Autodesk Fusion 360 part; units mm, degrees
(part 25 of 25)
sketch "Sketch2 (2)" plane through (0, 0, -3) normal (0, 0, -1) x (1, 0, 0) in component "grub screw"
  circle A0 centre (0, 0) radius 1.3
  line L0 (0.6928, 0.4) -> (0, 0.8)
  line L1 (0, 0.8) -> (-0.6928, 0.4)
  line L2 (-0.6928, 0.4) -> (-0.6928, -0.4)
  line L3 (-0.6928, -0.4) -> (0, -0.8)
  line L4 (0, -0.8) -> (0.6928, -0.4)
  line L5 (0.6928, -0.4) -> (0.6928, 0.4)
  dimension "d29" = 0.8
  constraint coincident A0.centre origin
  constraint vertical L5
  measures "d29" distance of L0.start A0.centre
extrude "Extrude2'" cut sketch "Sketch2 (2)" against normal blind 1.478 contours L0 L1 L2 L3 L4 L5 bodies 2 in component "grub screw"
sketch "Sketch1 (3)" plane through (0, 0, 11) normal (0, 0, 1) x (-1, 0, 0) in component "hex nut"
  circle A0 centre (0, 0) radius 0.875
  line L0 (0.6569, -2.1537) -> (2.1936, -0.5079)
  line L1 (2.1936, -0.5079) -> (1.5367, 1.6458)
  line L2 (1.5367, 1.6458) -> (-0.6569, 2.1537)
  line L3 (-0.6569, 2.1537) -> (-2.1936, 0.5079)
  line L4 (-2.1936, 0.5079) -> (-1.5367, -1.6458)
  line L5 (-1.5367, -1.6458) -> (0.6569, -2.1537)
  dimension "d32" = 1.95
  constraint coincident A0.centre origin
  measures "d32" distance of A0.centre L5
extrude "Extrude1''" add sketch "Sketch1 (3)" along normal blind 1.7 separate body makes body 3 in component "hex nut"
fillet "Fillet1" radius 0.494 6 edges at (0.6569, -2.1537, 11.85) (-1.5367, -1.6458, 11.85) (-2.1936, 0.5079, 11.85) (-0.6569, 2.1537, 11.85) (1.5367, 1.6458, 11.85) (2.1936, -0.5079, 11.85) on bodies 3 in component "hex nut"
fillet "Fillet1" radius 0.222 11 edges at (1.4253, -1.3308, 12.7) (-0.4399, -1.8997, 12.7) (-1.8652, -0.5689, 12.7) (-1.4253, 1.3308, 12.7) (0.4399, 1.8997, 12.7) (0.4399, 1.8997, 11) (-1.4253, 1.3308, 11) (-1.8652, -0.5689, 11) (-0.4399, -1.8997, 11) (1.4253, -1.3308, 11) (1.8652, 0.5689, 12.7) on bodies 3 in component "hex nut"
thread "Thread1" "ISO Metric profile 1.8 M1.8x0.35 6g" major diameter 1.7385 minor diameter 1.3386 pitch 0.35 angle 60 resizes the face on face at (-0.8739, 0.0436, 9) on bodies 1 in component "push rod connector"
thread "Thread1'" "ISO Metric profile 2.6 M2.6x0.45 6g" major diameter 2.53 minor diameter 2.0162 pitch 0.45 angle 60 resizes the face on face at (1.2935, 0.1294, -1.4667) on bodies 2 in component "grub screw"
thread "Thread2" "ISO Metric profile 2.5 M2.5x0.45 6H" major diameter 2.58 minor diameter 2.0755 pitch 0.45 angle 60 resizes the face on face at (-1.0349, -0.7868, 2.0472) on bodies 1 in component "push rod connector"
thread "Thread1''" "ISO Metric profile 1.7 M1.7x0.35 6H" major diameter 1.7678 minor diameter 1.3711 pitch 0.35 angle 60 resizes the face on face at (-0.8707, 0.0871, 11.5667) on bodies 3 in component "hex nut"
component "push rod connector" placed x (1, 0, 0) y (0, 1, 0) z (0, 0, 1) at (0, 0, 0)
component "grub screw" placed x (1, 0, 0) y (0, 1, 0) z (0, 0, 1) at (0, 0, 0)
component "hex nut" placed x (1, 0, 0) y (0, 1, 0) z (0, 0, 1) at (0, 0, 0)
equation "d29 = 1.6 mm / 2"
equation "d32 = 3.9 mm / 2"
